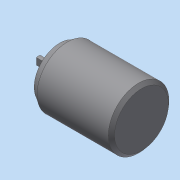
# Autodesk Inventor part: motor
Saved by Autodesk Inventor 2017 (Build 210142000, 142)
## iProperties
Created: 2016-01-05
Part Number: motor
Material: Generic
Document SubType Name: Modeling
Designer: JoshuaYuan
Density: 1 g/cm^3
Appearance: Default
Author: JoshuaYuan
Autodesk Inventor part; units mm, degrees
ref_plane "YZ Plane" through (0, 0, 0) normal (1, 0, 0) x (0, 1, 0)
ref_plane "XZ Plane" through (0, 0, 0) normal (0, 1, 0) x (-1, 0, 0)
sketch "Sketch1" plane through (0, 0, 0) normal (0, 0, 1) x (1, 0, 0)
  line L0 (0, 0) -> (0, -4)
  line L1 (0, -4) -> (22, -4)
  line L2 (22, -4) -> (22, -26.5)
  line L3 (22, -26.5) -> (30, -31.5)
  line L4 (30, -31.5) -> (104, -31.5)
  line L5 (104, -31.5) -> (107, -28)
  line L6 (107, -28) -> (107, 0)
  line L7 (-21.4, 0) -> (128.4, 0) projected
  line L8 (0, -37.8) -> (0, 6.3) projected
  line L9 (107, 0) -> (0, 0)
  dimension "d7" = 22.5
  dimension "d9" = 8
  dimension "d10" = 74
  dimension "d14" = 4
  dimension "d16" = 31.5
  dimension "d17" = 28
  dimension "d18" = 22
  dimension "d40" = 85
  constraints: 17 end point, 2 horizontal, 2 perpendicular, 1 collinear, 1 parallel, 1 vertical, 1 other
  measures "d7" distance of L1.end L2.end
  measures "d9" distance from line of L3.end L2
  measures "d10" distance of L3.end L4.end
  measures "d14" distance of L0.start L0.end
  measures "d16" distance between parallel lines of L9 L4
  measures "d17" distance of L5.end L6.end
  measures "d18" distance of L0.end L1.end
  measures "d40" distance between parallel lines of L6 L2
revolve "motor body" add sketch "Sketch1" angle 360 about axis through (-10, 0, 0) along (1, 0, 0)
sketch "Sketch4" plane through (0, 0, 0) normal (-1, 0, 0) x (0, 0, 1)
  circle A0 centre (0, 0) radius 4
  circle A1 centre (0, 0) radius 4 projected
  line L0 (2.0699, 3.4228) -> (2.0699, -3.4228)
  line L1 (0, -44.1) -> (0, 44.1) projected
  constraints: 4 point on circle, 2 end point, 1 centre point, 1 coincident, 1 parallel
extrude "axis slot" cut sketch "Sketch4" against normal blind 25 contours A0 L0
sketch "Sketch5" plane through (22, 0, 0) normal (-1, 0, 0) x (0, 0, 1)
  circle A0 centre (15.5, 15.5) radius 1.5875
  line L0 (0, -44.1) -> (0, 44.1) projected
  line L1 (-44.1, 0) -> (44.1, 0) projected
  circle A1 centre (15.5, -15.5) radius 1.5875
  circle A2 centre (-15.5, 15.5) radius 1.5875
  circle A3 centre (-15.5, -15.5) radius 1.5875
  point P0 (0, 0)
  dimension "d22" = 3.175
  dimension "d25" = 31
  dimension "d28" = 31
  dimension "d31" = 15.5
  dimension "d32" = 15.5
  constraints: 4 centre point, 1 horizontal, 1 vertical, 6 other
  measures "d22" diameter of A0
  measures "d25" distance of A0.centre A1.centre
  measures "d28" distance of A0.centre A2.centre
  measures "d31" horizontal distance of point (0, 0) A0.centre
  measures "d32" horizontal distance of point (0, 0) A0.centre
extrude "mounting holes" cut sketch "Sketch5" against normal blind 4
ref_plane "Work Plane1" through (67, 0, -31.5) normal (0, 0, 1) x (1, 0, 0)
sketch "Sketch6" plane through (67, 0, -31.5) normal (0, 0, 1) x (1, 0, 0)
  line L0 (-41.25, 10) -> (-41.25, -10) construction
  line L1 (-44, 10) -> (-44, -10)
  line L2 (-38.5, -10) -> (-38.5, 10)
  arc A0 (-38.5, 10) -> (-44, 10) centre (-41.25, 10) ccw
  arc A1 (-44, -10) -> (-38.5, -10) centre (-41.25, -10) ccw
  line L3 (-45, 26.5) -> (-45, -26.5) projected
  line L4 (-37, 31.5) -> (-37, -31.5) projected
  line L5 (-92, 0) -> (62, 0) projected
  point P0 (-67, 0)
  point P1 (-41.25, 0)
  dimension "d35" = 20
  dimension "d36" = 5.5
  dimension "d37" = 1.5
  constraints: 8 end point, 4 point on circle, 4 tangent, 2 centre point, 1 midpoint, 1 parallel, 1 point on line, 1 vertical
  measures "d35" distance of L0.end L0.start
  measures "d36" distance between parallel lines of L1 L2
  measures "d37" distance between parallel lines of L2 L4
extrude "cable hole" cut sketch "Sketch6" along normal blind 10
body "Solid2"
